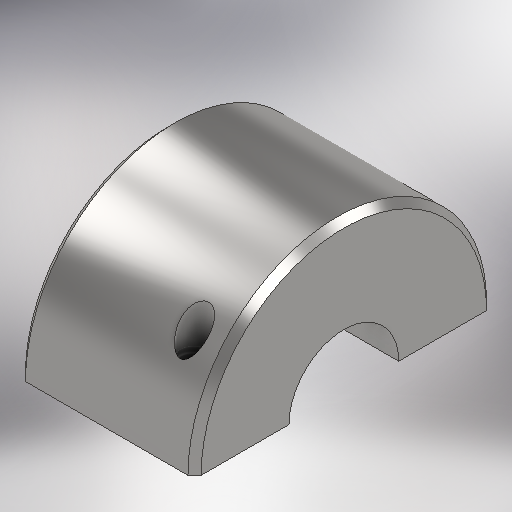
# Autodesk Inventor part: probe-cover
Saved by Autodesk Inventor 2026 (Build 300175050, 175E)
## iProperties
Created: 2025-10-27
Part Number: probe-cover
Material: ステンレス鋼
Document SubType Name: Modeling
Designer: jin20
Density: 8 g/cm^3
Appearance: 半つや出し
Author: jin20
Autodesk Inventor part; units mm, degrees
ref_plane "YZ Plane" through (0, 0, 0) normal (1, 0, 0) x (0, 1, 0)
ref_plane "XZ Plane" through (0, 0, 0) normal (0, 1, 0) x (-1, 0, 0)
ref_plane "XY Plane" through (0, 0, 0) normal (0, 0, 1) x (1, 0, 0)
sketch "スケッチ1" plane through (0, 0, 0) normal (0, 0, 1) x (1, 0, 0)
  line L0 (0, 0) -> (0, 6.25) construction
  line L1 (0, 6.25) -> (-10, 6.25)
  line L2 (-10, 6.25) -> (-10, 17)
  line L3 (-10, 17) -> (0, 17)
  line L4 (0, 6.25) -> (10, 6.25)
  line L5 (10, 6.25) -> (10, 17)
  line L6 (10, 17) -> (0, 17)
  line L7 (-14, 0) -> (14, 0) projected
  dimension "d0" = 6.25
  dimension "d1" = 10
  dimension "d2" = 10.75
  constraints: 14 end point, 1 horizontal, 1 parallel, 1 perpendicular, 1 vertical
  measures "d0" distance of L0.start L0.end
  measures "d1" distance of L2.end L3.end
  measures "d2" distance of L1.end L2.end
revolve "回転1" add sketch "スケッチ1" angle 180 mid plane about axis through (-10, 0, 0) along (1, 0, 0)
sketch "スケッチ2" plane through (-10, 0, 17) normal (0, -1, 0) x (1, 0, 0)
  line L0 (20, 0) -> (0, 0) projected
  line L1 (20, -10.75) -> (20, 0) projected
  point P0 (10, -17)
  point P1 (16, -4)
  dimension "d4" = 4
  dimension "d5" = 4
  measures "d4" distance from line of L0 point (16, -4)
  measures "d5" distance from line of L1 point (16, -4)
hole "穴1" at (6, 0, 13) direction (0, 1, 0) diameter 3.242 end through all thread size "M4x0.7" class "6H" standard "ANSI Metric M Profile"
mirror "ミラー1" about plane through (0, 0, 0) normal (0, 0, 1) of "穴1"
sketch "スケッチ3" plane through (-10, 0, -17) normal (-1, 0, 0) x (0, 0, 1)
  circle A0 centre (17, 0) radius 15.5
  dimension "d16" = 31
  constraints: 1 centre point, 1 coincident
  measures "d16" diameter of A0
extrude "押し出し1" cut sketch "スケッチ3" against normal blind 12
chamfer "面取り2" distance 0.75 angle 45 2 edges at (10, 17, 0) (-10, 17, 0)
